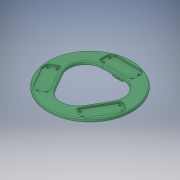
# Autodesk Inventor part: Stewart-Plate-inside
Saved by Autodesk Inventor 2018.2 (Build 222227000, 227)
## iProperties
Created: 2018-02-18
Part Number: Stewart-Plate-inside
Material: Generisch
Document SubType Name: Modeling
Designer: JochenAlt
Density: 1 g/cm^3
Appearance: Vorgabe
Author: JochenAlt
Autodesk Inventor part; units mm, degrees
ref_plane "YZ Plane" through (0, 0, 0) normal (1, 0, 0) x (0, 1, 0)
ref_plane "XZ Plane" through (0, 0, 0) normal (0, 1, 0) x (-1, 0, 0)
ref_plane "XY Plane" through (0, 0, 0) normal (0, 0, 1) x (1, 0, 0)
sketch "Skizze1" plane through (0, 0, 0) normal (0, 0, 1) x (1, 0, 0)
  line L0 (-56, 0) -> (56, 0) construction
  circle A0 centre (0, 0) radius 40
  line L1 (-8, 36) -> (8, 36)
  line L2 (8, 36) -> (8, 33)
  line L3 (8, 33) -> (-8, 33)
  line L4 (-8, 33) -> (-8, 36)
  line L5 (1.5, 33) -> (-1.5, 33)
  line L6 (-1.5, 33) -> (-1.5, 28)
  line L7 (-1.5, 28) -> (1.5, 28)
  line L8 (1.5, 28) -> (1.5, 33)
  circle A1 centre (0, 0) radius 7.5
  dimension "d9" = 80
  dimension "d10" = 3
  dimension "d11" = 33
  dimension "d14" = 16
  dimension "d23" = 5
  dimension "d62" = 15
  constraints: 16 end point, 4 parallel, 3 perpendicular, 2 centre point, 2 horizontal, 1 coincident, 1 midpoint, 1 point on line
  measures "d9" diameter of A0
  measures "d10" distance between parallel lines of L3 L1
  measures "d11" distance from line of L3 A0.centre
  measures "d14" distance between parallel lines of L2 L4
  measures "d23" distance between parallel lines of L3 L7
  measures "d62" diameter of A1
extrude "Extrusion3" add sketch "Skizze1" against normal blind 7 contours L1 L2 L3 L4 | L3 L8 L7 L6
fillet "Rundung1" radius 4 2 edges at (-8, 34.5, -7) (8, 34.5, -7)
sketch "Skizze2" plane through (-8, 36, 0) normal (0, 1, 0) x (1, 0, 0)
  circle A0 centre (3, 4) radius 1.1
  circle A1 centre (13, 4) radius 1.1
  line L0 (8, 0) -> (8, 7) construction
  line L1 (43, 0) -> (-27, 0) construction
  line L2 (-1.6221, 4) -> (19.0112, 4) construction
  line L3 (4, 7) -> (12, 7) construction
  line L4 (0, 0) -> (0, 3) projected
  dimension "d16" = 2.2
  dimension "d20" = 3
  dimension "d21" = 3
  constraints: 4 end point, 2 centre point, 1 equal radius, 1 horizontal, 1 midpoint, 1 point on line, 1 symmetric about line, 1 vertical
  measures "d16" diameter of A0
  measures "d20" distance between parallel lines of L3 L2
  measures "d21" distance from line of L4 A0.centre
extrude "Extrusion4" cut sketch "Skizze2" against normal up to next
chamfer "Fase1" distance 5 distance2 7 1 edges at (0, 28, -7) measured on face at (0, 28.5, -7)
pattern_circular "Runde Anordnung1" count 3 over 360 about axis through (0, 0, -10) along (0, 0, 1) of "Extrusion3", "Extrusion4", "Fase1", "Rundung1"
sketch "Skizze3" plane through (0, 0, 0) normal (0, 0, 1) x (1, 0, 0)
  line L0 (-11.9, 45.3) -> (-0.25, 45.3) construction
  line L1 (-0.25, 45.3) -> (-0.25, 30.3) construction
  line L2 (-0.25, 30.3) -> (-11.9, 30.3) construction
  line L3 (-11.9, 30.3) -> (-11.9, 45.3) construction
  line L4 (0.25, 45.3) -> (11.9, 45.3) construction
  line L5 (11.9, 45.3) -> (11.9, 30.3) construction
  line L6 (11.9, 30.3) -> (0.25, 30.3) construction
  line L7 (0.25, 30.3) -> (0.25, 45.3) construction
  line L8 (0, 70.94) -> (0, -77.1567) construction
  line L9 (-11.9, 31.4) -> (11.9, 31.4) construction
  line L10 (-11.9, 33.4) -> (11.9, 33.4) construction
  line L11 (-12.2, 45.6) -> (12.2, 45.6)
  line L12 (12.2, 45.6) -> (12.2, 30)
  line L13 (12.2, 30) -> (-12.2, 30)
  line L14 (-12.2, 30) -> (-12.2, 45.6)
  line L15 (-12.2, 31.1) -> (12.2, 31.1)
  line L16 (-12.2, 33.7) -> (12.2, 33.7)
  line L17 (-9.075, 43.3) -> (-9.075, 41.3) construction
  line L18 (-3.075, 43.3) -> (-3.075, 41.3) construction
  line L19 (3.075, 43.3) -> (3.075, 41.3) construction
  line L20 (9.075, 43.3) -> (9.075, 41.3) construction
  line L21 (6.075, 44.3) -> (6.075, 30.3) construction
  line L22 (-8.075, 44.3) -> (-4.075, 44.3) construction
  line L23 (-8.075, 40.3) -> (-4.075, 40.3) construction
  line L24 (4.075, 44.3) -> (8.075, 44.3) construction
  line L25 (4.075, 40.3) -> (8.075, 40.3) construction
  arc A0 (-8.075, 44.3) -> (-9.075, 43.3) centre (-8.075, 43.3) ccw construction
  arc A1 (-3.075, 43.3) -> (-4.075, 44.3) centre (-4.075, 43.3) ccw construction
  arc A2 (-4.075, 40.3) -> (-3.075, 41.3) centre (-4.075, 41.3) ccw construction
  arc A3 (-9.075, 41.3) -> (-8.075, 40.3) centre (-8.075, 41.3) ccw construction
  arc A4 (3.075, 41.3) -> (4.075, 40.3) centre (4.075, 41.3) ccw construction
  arc A5 (4.075, 44.3) -> (3.075, 43.3) centre (4.075, 43.3) ccw construction
  arc A6 (9.075, 43.3) -> (8.075, 44.3) centre (8.075, 43.3) ccw construction
  arc A7 (8.075, 40.3) -> (9.075, 41.3) centre (8.075, 41.3) ccw construction
  line L26 (-6.075, 45.3) -> (-6.075, 30.3) construction
  line L27 (-12.2, 30) -> (-12.2, 29) construction
  line L28 (12.2, 45.6) -> (14.2, 45.6)
  line L29 (20.2, 40.5585) -> (20.2, 33)
  line L30 (17.2, 30) -> (12.2, 30)
  line L31 (12.2, 30) -> (12.2, 45.6)
  line L32 (-12.2, 45.6) -> (-14.2, 45.6)
  line L33 (-20.2, 40.5585) -> (-20.2, 33)
  line L34 (-17.2, 30) -> (-12.2, 30)
  line L35 (-12.2, 30) -> (-12.2, 45.6)
  arc A8 (-20.2, 33) -> (-17.2, 30) centre (-17.2, 33) ccw
  arc A9 (17.2, 30) -> (20.2, 33) centre (17.2, 33) ccw
  circle A10 centre (17.2, 41) radius 1.3
  circle A11 centre (17.2, 33) radius 1.3
  circle A12 centre (-17.2, 41) radius 1.3
  circle A13 centre (-17.2, 33) radius 1.3
  line L36 (14.2, 45.6) -> (14.2, 30)
  line L37 (-14.2, 45.6) -> (-14.2, 30)
  circle A14 centre (0, 0) radius 40 construction
  line L38 (14.7, 45.466) -> (18.7, 43.1566)
  arc A15 (14.7, 45.466) -> (14.2, 45.6) centre (14.2, 44.6) ccw
  arc A16 (20.2, 40.5585) -> (18.7, 43.1566) centre (17.2, 40.5585) ccw
  line L39 (-14.7, 45.466) -> (-18.7, 43.1566)
  arc A17 (-18.7, 43.1566) -> (-20.2, 40.5585) centre (-17.2, 40.5585) ccw
  arc A18 (-14.2, 45.6) -> (-14.7, 45.466) centre (-14.2, 44.6) ccw
  circle A19 centre (0, 0) radius 49.7834
  line L40 (17.2, 33) -> (17.2, 41) construction
  line L41 (12.1244, 27) -> (-12.1244, 27)
  line L42 (-29.4449, -3) -> (-17.3205, -24)
  line L43 (29.4449, -3) -> (17.3205, -24)
  line L44 (-29.4449, 17) -> (23.3827, -13.5) construction
  line L45 (46.7654, 27) -> (-23.3827, -13.5) construction
  arc A20 (29.4449, -3) -> (12.1244, 27) centre (12.1244, 7) ccw
  arc A21 (-12.1244, 27) -> (-29.4449, -3) centre (-12.1244, 7) ccw
  arc A22 (-17.3205, -24) -> (17.3205, -24) centre (0, -14) ccw
  line L46 (-14.7, 45.466) -> (-15.3153, 47.369) construction
  point P0 (20.2, 42.2906)
  point P1 (-46.7654, 27)
  point P2 (0, -54)
  dimension "d36" = 11.65
  dimension "d37" = 0.5
  dimension "d38" = 15
  dimension "d42" = 2
  dimension "d43" = 0.3
  dimension "d44" = 0.3
  dimension "d45" = 0.3
  dimension "d46" = 0.3
  dimension "d47" = 0.3
  dimension "d48" = 0.3
  dimension "d51" = 6
  dimension "d52" = 1
  dimension "d53" = 5
  dimension "d54" = 1
  dimension "d61" = 1
  dimension "d68" = 2.6
  dimension "d70" = 2
  dimension "d71" = 8
  dimension "d84" = 3
  dimension "d86" = 1
  dimension "d88" = 60
  dimension "d133" = 1.1
  dimension "d136" = 8
  dimension "d139" = 30
  dimension "d140" = 60
  dimension "d141" = 20
  dimension "d143" = 3
  dimension "d144" = 20
  dimension "d145" = 2
  constraints: 94 end point, 35 point on circle, 33 tangent, 21 centre point, 21 point on line, 20 perpendicular, 15 equal radius, 12 parallel, 7 collinear, 6 horizontal, 6 midpoint, 3 coincident, 2 symmetric about line, 1 line through centre, 1 vertical, 12 other
  measures "d36" distance between parallel lines of L5 L7
  measures "d37" distance between parallel lines of L7 L1
  measures "d38" distance between parallel lines of L4 L6
  measures "d42" distance between parallel lines of L9 L10
  measures "d43" distance between parallel lines of L4 L11
  measures "d44" distance between parallel lines of L5 L12
  measures "d45" distance between parallel lines of L13 L6
  measures "d46" distance between parallel lines of L3 L14
  measures "d47" distance between parallel lines of L10 L16
  measures "d48" distance between parallel lines of L15 L9
  measures "d51" distance between parallel lines of L20 L19
  measures "d52" distance between parallel lines of L4 L24
  measures "d53" distance between parallel lines of L25 L4
  measures "d54" radius of A0
  measures "d61" distance of L13.end L27.end
  measures "d68" diameter of A10
  measures "d70" distance between parallel lines of L12 L36
  measures "d71" distance between parallel lines of L29 L12
  measures "d84" radius of A8
  measures "d86" radius of A15
  measures "d88" angle of L36 L38
  measures "d133" distance between parallel lines of L9 L6
  measures "d136" distance of A9.centre L40.end
  measures "d139" distance from line of point (0, 0) L13
  measures "d140" angle of L43 L41
  measures "d141" radius of A20
  measures "d143" distance between parallel lines of L13 L41
  measures "d144" radius of A22
  measures "d145" distance of L39.start L46.end
extrude "Extrusion9" add sketch "Skizze3" along normal blind 4 contours L11 L12 L16 L14 | L14 L34 L37 L32 | L28 L36 L30 L12 | L16 L12 L15 L14 | L37 L34 A8 L33 A17 L39 A18 | A15 L38 A16 L29 A9 L30 L36 | L15 L12 L13 L14 | A10 | A11 | A12 | A13 | A19
extrude "Extrusion6" add sketch "Skizze3" against normal blind 2 from surface at 4 separate body contours L11 L12 L16 L14 | L14 L34 L37 L32 | L28 L36 L30 L12 | L16 L12 L15 L14 | L37 L34 A8 L33 A17 L39 A18 | A15 L38 A16 L29 A9 L30 L36 | L15 L12 L13 L14 | A10 | A11 | A12 | A13
extrude "Extrusion10" add sketch "Skizze3" along normal blind 4 contours A10 | A11 | A12 | A13 bodies 2
pattern_circular "Runde Anordnung2" count 3 over 360 about axis through (0, 0, -10) along (0, 0, 1) of "Extrusion6", "Extrusion10" bodies 2
combine bodies "Kombinieren3" operation type subtract main body 1 bodies to subtract 2
fillet "Rundung4" radius 1 14 edges at (23.3827, -13.5, 4) (0, -34, 4) (-23.3827, -13.5, 4) (-29.4449, 17, 4) (0, 27, 4) (29.4449, 17, 4) (-49.7834, 0, 4) (-49.7834, 0, 0) (29.4449, 17, 0) (0, 27, 0) (23.3827, -13.5, 0) (0, -34, 0) (-23.3827, -13.5, 0) (-29.4449, 17, 0)
equation "\"d21\" = d20"
equation "\"d44\" = d43"
equation "\"d45\" = d43"
equation "\"d46\" = d43"
equation "\"d47\" = d43"
equation "\"d48\" = d43"
